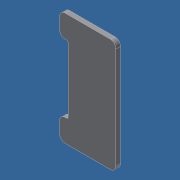
# Autodesk Inventor part: Pièce1
Saved by Autodesk Inventor 2015 SP2 (Build 190223200, 223)
## iProperties
Created: 2018-05-24
Part Number: Pièce1
Material: Générique
Document SubType Name: Modeling
Designer: Pierre-Olivier.SANDO
Density: 1 g/cm^3
Appearance: Par défaut
Author: Pierre-Olivier.SANDO
Autodesk Inventor part; units mm, degrees
ref_plane "YZ Plane" through (0, 0, 0) normal (1, 0, 0) x (0, 1, 0)
ref_plane "XZ Plane" through (0, 0, 0) normal (0, 1, 0) x (-1, 0, 0)
ref_plane "XY Plane" through (0, 0, 0) normal (0, 0, 1) x (1, 0, 0)
sketch "Esquisse1" plane through (0, 0, 0) normal (0, 1, 0) x (-1, 0, 0)
  line L0 (0, 0) -> (-100, 0)
  line L1 (-100, 0) -> (-100, 200)
  line L2 (-100, 200) -> (0, 200)
  line L3 (0, 200) -> (0, 0)
  dimension "d0" = 100
  dimension "d1" = 200
  constraints: 8 end point, 2 parallel, 1 horizontal, 1 perpendicular
  measures "d0" distance of L1.end L2.end
  measures "d1" distance of L0.end L1.end
extrude "Extrusion1" add sketch "Esquisse1" along normal blind 8
fillet "Congé1" radius 10 1 edges at (100, 4, 0)
fillet "Congé2" radius 10 1 edges at (100, 4, 200)
fillet "Congé3" radius 10 1 edges at (0, 4, 0)
fillet "Congé4" radius 10 1 edges at (0, 4, 200)
sketch "Esquisse2" plane through (0, 8, 0) normal (0, 1, 0) x (1, 0, 0)
  line L0 (0, -40) -> (15, -40)
  line L1 (15, -40) -> (15, -160)
  line L2 (15, -160) -> (0, -160)
  line L3 (0, -160) -> (0, -40)
  line L4 (0, -190) -> (0, -10) projected
  line L5 (0, -40) -> (99.7928, -40)
  line L6 (0, -160) -> (99.7928, -160)
  line L7 (90, 0) -> (10, 0) projected
  line L8 (10, -200) -> (90, -200) projected
  line L9 (0, -10) -> (0, -190) projected
  point P0 (0, 0)
  dimension "d9" = 15
  dimension "d10" = 40
  dimension "d16" = 40
  constraints: 12 end point, 3 collinear, 3 horizontal, 3 parallel, 2 perpendicular, 2 point on line
  measures "d9" distance of L0.start L0.end
  measures "d10" distance between parallel lines of L5 L7
  measures "d16" distance between parallel lines of L8 L6
extrude "Extrusion2" cut sketch "Esquisse2" against normal blind 8
fillet "Congé5" radius 10 1 edges at (0, 4, 40)
fillet "Congé6" radius 10 1 edges at (0, 4, 160)
fillet "Congé7" radius 2 1 edges at (15, 4, 40)
fillet "Congé8" radius 2 1 edges at (15, 4, 160)
equation "\"d16\" = d10"
